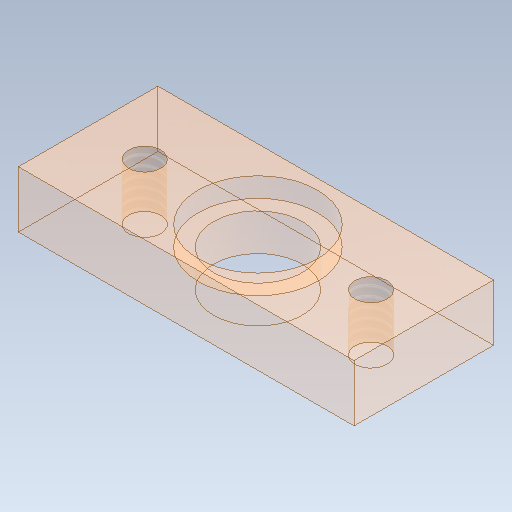
# Autodesk Inventor part: main_manifold_cover_1v
Saved by Autodesk Inventor 2020.5 (Build 245400000, 400)
## iProperties
Created: 2021-06-11
Part Number: main_manifold_cover_1v
Material: Generic
Document SubType Name: Modeling
Designer: shann
Density: 1 g/cm^3
Appearance: Clear - Yellow(1)
connScrews:z:distFromFront: 0.225 in
a_mainManifoldCover:y:height: 0.150 in
x_d0: 1.000 ul
x_e1: 0.00 deg
flowSensor:throughHole:diameter: 0.235 in
MMCscrews:z:distFromFront: 0.180 in
MMCscrews:distFromFront: 0.185 in
MMCscrew:dist_from_back: 0.185 in
MMCscrew:dist_from_side:L: 0.150 in
flowSensor:oring:OD: 0.316 in
flowSensor:oring:depth: 0.052 in
MMCscrew:dist_from_side:R: 0.140 in
screws:4_40:MMC:thread:depth: 0.224 in
Author: shann
Autodesk Inventor part; units mm, degrees
ref_plane "YZ Plane" through (0, 0, 0) normal (1, 0, 0) x (0, 1, 0)
ref_plane "XZ Plane" through (0, 0, 0) normal (0, 1, 0) x (-1, 0, 0)
ref_plane "XY Plane" through (0, 0, 0) normal (0, 0, 1) x (1, 0, 0)
derived "main_manifold_8v.ipt"
sketch "Sketch:MM: flow sensor" plane through (0, 0, -27.94) normal (0, -1, 0) x (1, 0, 0)
  line L0 (19.2278, 23.241) -> (22.6822, 23.241)
  line L1 (49.7078, 23.241) -> (53.1622, 23.241)
  line L2 (110.6678, 23.241) -> (114.1222, 23.241)
  line L3 (80.1878, 23.241) -> (83.6422, 23.241)
  line L4 (141.1478, 23.241) -> (144.6022, 23.241)
  line L5 (171.6278, 23.241) -> (175.0822, 23.241)
  line L6 (202.1078, 23.241) -> (205.5622, 23.241)
  line L7 (232.5878, 23.241) -> (236.0422, 23.241)
  line L8 (0, 27.94) -> (247.65, 27.94)
  point P0 (20.955, 23.241)
  point P1 (51.435, 23.241)
  point P2 (51.435, 23.241)
  point P3 (20.955, 23.241)
  point P4 (81.915, 23.241)
  point P5 (112.395, 23.241)
  point P6 (81.915, 23.241)
  point P7 (112.395, 23.241)
  point P8 (142.875, 23.241)
  point P9 (173.355, 23.241)
  point P10 (203.835, 23.241)
  point P11 (234.315, 23.241)
  point P12 (142.875, 23.241)
  point P13 (173.355, 23.241)
  point P14 (203.835, 23.241)
  point P15 (234.315, 23.241)
sketch "Sketch:MM: MMC screws" plane through (0, 20.32, 0) normal (0, 1, 0) x (1, 0, 0)
  line L0 (0, 0) -> (0, 27.94)
  line L1 (43.815, 4.699) -> (59.055, 4.699) construction
  line L2 (0, 0) -> (247.65, 0)
  line L3 (13.335, 4.699) -> (28.575, 4.699) construction
  line L4 (74.295, 4.699) -> (89.535, 4.699) construction
  line L5 (104.775, 4.699) -> (120.015, 4.699) construction
  line L6 (135.255, 4.699) -> (150.495, 4.699) construction
  line L7 (165.735, 4.699) -> (180.975, 4.699) construction
  line L8 (196.215, 4.699) -> (211.455, 4.699) construction
  line L9 (226.695, 4.699) -> (241.935, 4.699) construction
  point P0 (95.1312, 5.08)
  point P1 (20.955, 4.699)
  point P2 (112.395, 4.699)
  point P3 (51.435, 4.699)
  point P4 (81.915, 4.699)
  point P5 (0, 25.781)
  point P6 (0, 25.781)
  point P7 (0, 25.781)
  point P8 (142.875, 4.699)
  point P9 (173.355, 4.699)
  point P10 (203.835, 4.699)
  point P11 (234.315, 4.699)
  point P12 (125.6112, 5.08)
  point P13 (156.0912, 5.08)
  point P14 (186.5712, 5.08)
  point P15 (217.0512, 5.08)
  point P16 (244.1022, 5.08)
  point P17 (20.955, 4.699)
  point P18 (51.435, 4.699)
  point P19 (81.915, 4.699)
  point P20 (112.395, 4.699)
  point P21 (142.875, 4.699)
  point P22 (173.355, 4.699)
  point P23 (203.835, 4.699)
  point P24 (234.315, 4.699)
sketch "Sketch:MMC: base" plane through (0, 0, 0) normal (0, 1, 0) x (-1, 0, 0)
  line L0 (-9.525, -9.398) -> (-32.131, -9.398)
  line L1 (-32.131, -9.398) -> (-32.131, 0)
  line L2 (-32.131, 0) -> (-9.525, 0)
  line L3 (-9.525, 0) -> (-9.525, -9.398)
  point P0 (0, 0)
  point P1 (-43.815, -4.699)
  point P2 (-9.525, -4.699)
  point P3 (-13.335, -4.699)
  point P4 (-28.575, -4.699)
  constraints: 8 end point, 3 perpendicular, 1 horizontal alignment, 1 midpoint, 1 vertical, 3 other
extrude "Ex: base" add sketch "Sketch:MMC: base" against normal blind 3.81
hole "Hole: flowSensor" at (20.955, 0, -4.699) at (51.435, 0, -4.699) at (81.915, 0, -4.699) at (112.395, 0, -4.699) at (142.875, 0, -4.699) at (173.355, 0, -4.699) at (203.835, 0, -4.699) at (234.315, 0, -4.699) direction (0, -1, 0) diameter 5.969 end through all counterbore diameter 8.0264 counterbore depth 1.3208
hole "Hole: MMC screws" at (13.335, 0, -4.699) at (28.575, 0, -4.699) direction (0, -1, 0) diameter 2.1565 end through all thread size "4-40 UNC" class "2B" standard "ANSI Unified Screw Threads"
body "Solid1"
